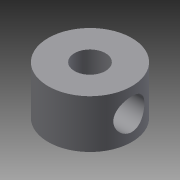
# Autodesk Inventor part: Axle hub with no cricle thing
Saved by Autodesk Inventor 2015 (Build 190159000, 159)
## iProperties
Created: 2014-12-01
Part Number: Axle hub with no cricle thing
Material: Generic
Document SubType Name: Modeling
Designer: lethcoec
Density: 1 g/cm^3
Appearance: Default
Author: lethcoec
Autodesk Inventor part; units mm, degrees
ref_plane "XZ Plane" through (0, 0, 0) normal (0, 1, 0) x (-1, 0, 0)
ref_plane "XY Plane" through (0, 0, 0) normal (0, 0, 1) x (1, 0, 0)
sketch "Sketch1" plane through (0, 0, 0) normal (0, 1, 0) x (-1, 0, 0)
  circle A0 centre (0, 0) radius 5.5182
  dimension "d0" = 11.0363
  constraints: 1 centre point, 1 coincident
  measures "d0" diameter of A0
extrude "Extrusion1" add sketch "Sketch1" along normal blind 6.3779
sketch "Sketch2" plane through (0, 6.3779, 0) normal (0, 1, 0) x (1, 0, 0)
  circle A0 centre (0, 0) radius 2.046
  dimension "d3" = 4.0919
  constraints: 1 centre point, 1 coincident
  measures "d3" diameter of A0
extrude "Extrusion2" cut sketch "Sketch2" against normal blind 11.1125
ref_plane "Work Plane1" through (5.5182, 0, 0) normal (1, 0, 0) x (0, 1, 0)
sketch "Sketch3" plane through (5.5182, 0, 0) normal (1, 0, 0) x (0, 1, 0)
  line L0 (6.3779, -5.5182) -> (6.3779, 5.5182) projected
  line L1 (6.3779, 0) -> (0, 0)
  circle A0 centre (3.189, 0) radius 2.0472
  dimension "d6" = 4.0945
  constraints: 2 end point, 2 midpoint, 1 centre point, 1 horizontal
  measures "d6" diameter of A0
extrude "Extrusion3" cut sketch "Sketch3" against normal blind 5.3975
body "Solid1"
